Autodesk Fusion 360 part; units mm, degrees
(part 2 of 2)
sketch "USB B" plane through (0, 0, 0) normal (0, 1, 0) x (1, 0, 0) in component "USB"
  line L0 (7.35, -2.05) -> (7.35, 2.05)
  arc A0 (7.35, 2.05) -> (5.75, 3.65) centre (5.75, 2.05) ccw
  line L1 (5.75, 3.65) -> (-5.75, 3.65)
  arc A1 (-5.75, 3.65) -> (-7.35, 2.05) centre (-5.75, 2.05) ccw
  line L2 (-7.35, 2.05) -> (-7.35, -2.05)
  arc A2 (-7.35, -2.05) -> (-5.75, -3.65) centre (-5.75, -2.05) ccw
  line L3 (-5.75, -3.65) -> (5.75, -3.65)
  arc A3 (5.75, -3.65) -> (7.35, -2.05) centre (5.75, -2.05) ccw
  line L4 (0, 0) -> (-15, 0) construction
  circle A4 centre (-15, 0) radius 1.8
  circle A5 centre (15, 0) radius 1.8
  line L5 (7.35, 3.65) -> (-7.35, -3.65) construction
  line L6 (-7.35, 3.65) -> (7.35, -3.65) construction
  line L7 (20, 7.5) -> (-20, 7.5)
  line L8 (-20, 7.5) -> (-20, -7.5)
  line L9 (-20, -7.5) -> (20, -7.5)
  line L10 (20, -7.5) -> (20, 7.5)
  line L11 (20, 7.5) -> (-20, -7.5) construction
  line L12 (-20, 7.5) -> (20, -7.5) construction
  line L13 (0, -7.5) -> (0, 0) construction
  dimension "d555" = 14.7
  dimension "d556" = 7.3
  dimension "d557" = 1.6
  dimension "d558" = 1.6
  dimension "d559" = 1.6
  dimension "d560" = 1.6
  dimension "d561" = 15
  dimension "d562" = 3.6
  dimension "d240" = 15
  dimension "d241" = 40
  constraint horizontal L1
  constraint perpendicular L1 L2
  constraint parallel L1 L3
  constraint parallel L0 L2
  constraint coincident L6.start L1
  constraint coincident L6.start L2
  constraint tangent L1 A1
  constraint tangent A1 L2
  constraint coincident L5.start L0
  constraint coincident L5.start L1
  constraint tangent L0 A0
  constraint tangent A0 L1
  constraint coincident L6.end L0
  constraint coincident L6.end L3
  constraint tangent L0 A3
  constraint tangent L3 A3
  constraint coincident L5.end L2
  constraint coincident L5.end L3
  constraint tangent L2 A2
  constraint tangent A2 L3
  constraint perpendicular L2 L4
  constraint coincident L4.end A4.centre
  constraint horizontal L7
  constraint perpendicular L7 L8
  constraint parallel L7 L9
  constraint parallel L8 L10
  constraint coincident L11 L4.start
  constraint coincident L12 L4.start
  constraint coincident L4.start L13.end
  constraint midpoint L9 L13.start
  constraint symmetric A4 A5 L13
  measures "d555" distance of L5.end L6.end
  measures "d556" distance of L6.start L5.end
  measures "d557" radius of A1
  measures "d558" radius of A0
  measures "d559" radius of A3
  measures "d560" radius of A2
  measures "d561" distance of L4.end L4.start
  measures "d562" diameter of A4
  measures "d240" distance of L7.end L8.end
  measures "d241" distance of L8.end L9.end
sketch "RJ-45" plane through (0, 0, 0) normal (0, 1, 0) x (1, 0, 0) in component "Other Connectors"
  line L0 (0, -15.1) -> (0, 0)
  line L1 (0, 0) -> (17.8, 0)
  line L2 (17.8, 0) -> (17.8, -15.1)
  line L3 (17.8, -15.1) -> (0, -15.1)
  circle A0 centre (-4.6, -9.15) radius 1.675
  circle A1 centre (22.4, -9.15) radius 1.675
  line L4 (0, -15.1) -> (17.8, 0) construction
  line L5 (17.8, -15.1) -> (0, 0) construction
  line L6 (-4.6, -9.15) -> (22.4, -9.15) construction
  line L7 (8.9, -7.55) -> (8.9, -9.15) construction
  line L8 (26.4, 4.95) -> (-8.6, 4.95)
  line L9 (-8.6, 4.95) -> (-8.6, -20.05)
  line L10 (-8.6, -20.05) -> (26.4, -20.05)
  line L11 (26.4, -20.05) -> (26.4, 4.95)
  line L12 (26.4, 4.95) -> (-8.6, -20.05) construction
  line L13 (-8.6, 4.95) -> (26.4, -20.05) construction
  line L14 (8.9, -7.55) -> (14, -7.55) construction
  point P0 (8.9, -7.55)
  dimension "d596" = 3.35
  dimension "d597" = 3.35
  dimension "d244" = 1.6
  dimension "d245" = 15.1
  dimension "d246" = 17.8
  dimension "d247" = 27
  dimension "d248" = 35
  dimension "d249" = 25
  constraint coincident A0.centre L6.start
  constraint coincident A1.centre L6.end
  constraint perpendicular L2 L6
  constraint midpoint L5 P0
  constraint midpoint L6 L7.end
  constraint horizontal L8
  constraint perpendicular L8 L9
  constraint parallel L8 L10
  constraint parallel L9 L11
  constraint coincident L12 P0
  constraint coincident L13 P0
  constraint coincident P0 L7.start
  constraint perpendicular L7 L14
  constraint symmetric L8 L10 L14
  measures "d596" diameter of A0
  measures "d597" diameter of A1
  measures "d244" distance of P0 L7.end
  measures "d245" distance of L0.start L0.end
  measures "d246" distance of L2.end L0.start
  measures "d247" distance of A0.centre A1.centre
  measures "d248" distance of L9.end L10.end
  measures "d249" distance of L8.end L9.end
sketch "HDMI" plane through (0, 0, 0) normal (0, 1, 0) x (1, 0, 0) in component "Other Connectors"
  line L0 (-8.15, -3.0387) -> (-8.15, 1.8613)
  line L1 (-8.15, 1.8613) -> (-6.55, 1.8613)
  line L2 (-6.55, 1.8613) -> (-5.7382, 2.8326)
  line L3 (-5.7382, 2.8326) -> (0, 2.8326)
  line L4 (8.15, -3.0387) -> (-8.15, -3.0387)
  line L5 (8.15, -3.0387) -> (8.15, 1.8613)
  line L6 (8.15, 1.8613) -> (6.55, 1.8613)
  line L7 (6.55, 1.8613) -> (5.7382, 2.8326)
  line L8 (5.7382, 2.8326) -> (0, 2.8326)
  line L9 (0, 0) -> (13.25, 0) construction
  line L10 (0, 6) -> (0, -6) construction
  circle A0 centre (-13.25, 0) radius 1.8
  circle A1 centre (13.25, 0) radius 1.8
  line L11 (20, 6) -> (-20, 6)
  line L12 (-20, 6) -> (-20, -6)
  line L13 (-20, -6) -> (20, -6)
  line L14 (20, -6) -> (20, 6)
  dimension "d571" = 16.3
  dimension "d573" = 4.9
  dimension "d574" = 1.6
  dimension "d579" = 3.6
  dimension "d256" = 40
  dimension "d257" = 12
  constraint parallel L3 L4
  constraint coincident L3.end L10
  constraint coincident L9.end A1.centre
  constraint coincident L4.start L5
  constraint coincident L5.start L4
  constraint coincident L8.end L3
  constraint horizontal L9
  constraint horizontal L4
  constraint symmetric L10 A0 A1
  constraint symmetric L0 L5 L10
  constraint symmetric L2 L7 L10
  constraint symmetric L3 L8 L10
  constraint symmetric L10 L12 L14
  constraint symmetric L9 L11 L13
  measures "d571" distance of L4.start L0.start
  measures "d573" distance of L0.end L0.start
  measures "d574" distance of L0.end L1.end
  measures "d579" diameter of A1
  measures "d256" distance of L12.end L13.end
  measures "d257" distance of L12.end L11.end
sketch "40mm Fan Profile" plane through (0, 0, 0) normal (0, 1, 0) x (1, 0, 0) in component "Fans"
  circle A0 centre (0, 0) radius 19.5
  line L0 (16, 16) -> (-16, 16) construction
  line L1 (-16, 16) -> (-16, -16) construction
  line L2 (-16, -16) -> (16, -16) construction
  line L3 (16, -16) -> (16, 16) construction
  line L4 (16, 16) -> (-16, -16) construction
  line L5 (-16, 16) -> (16, -16) construction
  circle A1 centre (-16, 16) radius 1.8
  circle A2 centre (16, 16) radius 1.8
  circle A3 centre (-16, -16) radius 1.8
  circle A4 centre (16, -16) radius 1.8
  dimension "d258" = 39
  dimension "d259" = 32
  dimension "d260" = 32
  dimension "d261" = 3.6
  dimension "d262" = 3.6
  dimension "d263" = 3.6
  dimension "d264" = 3.6
  constraint coincident A0.centre origin
  constraint horizontal L0
  constraint perpendicular L0 L1
  constraint parallel L0 L2
  constraint parallel L1 L3
  constraint coincident L4 A0.centre
  constraint coincident L5 A0.centre
  constraint coincident L0.end L1.start
  constraint coincident L0.start L3.end
  constraint coincident L1.end L2.start
  constraint coincident L2.end L3.start
  measures "d258" diameter of A0
  measures "d259" distance of L1.end L2.end
  measures "d260" distance of L0.end L1.end
  measures "d261" diameter of A1
  measures "d262" diameter of A2
  measures "d263" diameter of A4
  measures "d264" diameter of A3
sketch "MF3 2R 14P" plane through (0, 0, 0) normal (0, 1, 0) x (1, 0, 0) in component "Molex Micro Fit 3"
  line L0 (-0.85, -4.975) -> (0.85, -3.575) construction
  line L1 (-11.075, 3.575) -> (11.075, -3.575) construction
  line L2 (0.85, -4.975) -> (-0.85, -3.575) construction
  line L3 (-13.25, 1.875) -> (13.25, -1.875) construction
  line L4 (-11.075, 3.575) -> (-11.075, -3.575) construction
  line L5 (0.85, -3.575) -> (11.075, -3.575)
  line L6 (11.075, 3.575) -> (-11.075, -3.575) construction
  line L7 (-0.85, -3.575) -> (-11.075, -3.575)
  line L8 (11.075, 3.575) -> (-11.075, 3.575)
  line L9 (0, -3.575) -> (0, -4.975) construction
  line L10 (-11.075, -3.575) -> (-11.075, -1.875)
  line L11 (0, -4.975) -> (0, 3.575) construction
  line L12 (14.75, 4.8) -> (14.75, -6.2)
  line L13 (13.25, 1.875) -> (-13.25, -1.875) construction
  line L14 (0.85, -4.975) -> (-0.85, -4.975)
  line L15 (-14.75, -6.2) -> (-14.75, 4.8)
  line L16 (-14.75, 4.8) -> (14.75, 4.8)
  line L17 (11.075, 1.875) -> (11.075, 3.575)
  line L18 (-11.075, -1.875) -> (-13.25, -1.875)
  line L19 (11.075, 1.875) -> (13.25, 1.875)
  line L20 (11.075, -1.875) -> (13.25, -1.875)
  line L21 (11.075, -3.575) -> (11.075, 3.575) construction
  line L22 (0.85, -3.575) -> (0.85, -4.975)
  line L23 (-13.25, 1.875) -> (-13.25, -1.875)
  line L24 (13.25, -1.875) -> (13.25, 1.875)
  line L25 (-11.075, 1.875) -> (-11.075, 3.575)
  line L26 (-0.85, -4.975) -> (-0.85, -3.575)
  line L27 (-13.25, 1.875) -> (-11.075, 1.875)
  line L28 (-11.075, -3.575) -> (11.075, -3.575) construction
  line L29 (13.25, 1.875) -> (-13.25, 1.875) construction
  line L30 (11.075, -3.575) -> (11.075, -1.875)
  line L31 (-13.25, -1.875) -> (13.25, -1.875) construction
  line L32 (-0.85, -3.575) -> (0.85, -3.575) construction
  line L33 (14.75, -6.2) -> (-14.75, -6.2)
  line L34 (14.75, -6.2) -> (-14.75, 4.8) construction
  line L35 (-14.75, -6.2) -> (14.75, 4.8) construction
  point P0 (-3, 0)
  point P1 (0, -0.7)
  point P2 (0, -4.275)
  dimension "d330" = 22.15
  dimension "d331" = 7.15
  dimension "d332" = 26.5
  dimension "d333" = 3.75
  dimension "d334" = 1.4
  dimension "d335" = 1.7
  dimension "d336" = 29.5
  dimension "d337" = 11
  constraint horizontal L8
  constraint perpendicular L4 L8
  constraint parallel L8 L28
  constraint parallel L4 L21
  constraint coincident origin L6
  constraint coincident origin L1
  constraint horizontal L29
  constraint perpendicular L23 L29
  constraint parallel L29 L31
  constraint parallel L23 L24
  constraint coincident origin L13
  constraint coincident origin L3
  constraint midpoint L9.start L28
  constraint perpendicular L9 L28
  constraint horizontal L14
  constraint perpendicular L14 L26
  constraint parallel L14 L32
  constraint parallel L22 L26
  constraint coincident P2 L2
  constraint coincident P2 L0
  constraint midpoint P2 L9
  constraint perpendicular L4 L7
  constraint coincident L10.end L31
  constraint coincident L10.end L4
  constraint coincident L25.start L29
  constraint coincident L25.start L4
  constraint coincident L17.start L29
  constraint coincident L17.start L21
  constraint coincident L20.start L21
  constraint coincident L20.start L31
  constraint midpoint L11.end L8
  constraint horizontal L33
  constraint perpendicular L15 L33
  constraint parallel L16 L33
  constraint parallel L12 L15
  constraint coincident P1 L34
  constraint coincident P1 L35
  constraint midpoint P1 L11
  measures "d330" distance of L4.end L1.end
  measures "d331" distance of L1.start L4.end
  measures "d332" distance of L13.end L3.end
  measures "d333" distance of L13.end L3.start
  measures "d334" distance of L9.start L9.end
  measures "d335" distance of L0.end L2.end
  measures "d336" distance of L15.start L12.end
  measures "d337" distance of L15.start L15.end
extrude "Extrude1" add sketch "MF3 1R 2P" along normal blind 1.8 makes body 1 in component "MF3 1R 2P"
extrude "Extrude1'" add sketch "MF3 1R 3P" along normal blind 1.8 separate body makes body 2 in component "MF3 1R 3P"
extrude "Extrude1''" add sketch "MF3 1R 4P" along normal blind 1.8 separate body makes body 3 in component "MF3 1R 4P"
extrude "Extrude1'''" add sketch "MF3 1R 5P" along normal blind 1.8 separate body makes body 4 in component "MF3 1R 5P"
extrude "Extrude1''''" add sketch "MF3 2R 2P" along normal blind 1.8 separate body makes body 5 in component "MF3 2R 2P"
extrude "Extrude1'''''" add sketch "MF3 2R 4P" along normal blind 1.8 separate body makes body 6 in component "MF3 2R 4P"
extrude "Extrude1''''''" add sketch "MF3 2R 6P" along normal blind 2.4 separate body makes body 7 in component "MF3 2R 6P"
extrude "Extrude1'''''''" add sketch "MF3 2R 8P" along normal blind 1.8 separate body makes body 8 in component "MF3 2R 8P"
extrude "Extrude1''''''''" add sketch "MF3 2R 10P" along normal blind 2.4 separate body makes body 9 in component "MF3 2R 10P"
extrude "Extrude1'''''''''" add sketch "MF3 2R 12P" along normal blind 2.4 separate body makes body 10 in component "MF3 2R 12P"
extrude "Extrude1''''''''''" add sketch "MF3 2R 14P" along normal blind 2.4 separate body makes body 11 in component "MF3 2R 14P"
extrude "Extrude1'''''''''''" add sketch "MF3 2R 16P" along normal blind 1.8 separate body makes body 12 in component "MF3 2R 16P"
sketch "USB Logo" plane through (0, 0, 0) normal (0, 1, 0) x (1, 0, 0) in component "USB"
  spline S0 degree 3 poles (-0.5083, -3.738) (-0.113, -4.1192) (0.5084, -4.4442) (1.1013, -4.4442) knots 0 0 0 0 1 1 1 1
  line L0 (1.1013, -4.4442) -> (3.2091, -4.4437)
  line L1 (3.2091, -4.4437) -> (3.2091, -5.3315)
  line L2 (3.2091, -5.3315) -> (5.8576, -5.3315)
  line L3 (5.8576, -5.3315) -> (5.8576, -2.6833)
  line L4 (5.8576, -2.6833) -> (3.2091, -2.6833)
  line L5 (3.2091, -2.6833) -> (3.2091, -3.5699)
  spline S1 degree 2 poles (3.2091, -3.5699) (2.6539, -3.5689) (1.0755, -3.5689) knots 0 0 0 1 1 1
  spline S2 degree 3 poles (1.0755, -3.5689) (0.7736, -3.562) (0.4799, -3.436) (0.2557, -3.2563) knots 0 0 0 0 1 1 1 1
  line L6 (0.2557, -3.2563) -> (-2.38, -0.4717)
  line L7 (-2.38, -0.4717) -> (7.8439, -0.4717)
  line L8 (7.8439, -0.4717) -> (7.8439, -1.5642)
  line L9 (7.8439, -1.5642) -> (10.4917, -0.0354)
  line L10 (10.4917, -0.0354) -> (7.8439, 1.4937)
  line L11 (7.8439, 1.4937) -> (7.8439, 0.403)
  line L12 (7.8439, 0.403) -> (-5.6896, 0.403)
  line L13 (-5.6896, 0.403) -> (-3.0545, 3.187)
  spline S3 degree 3 poles (-3.0545, 3.187) (-2.8302, 3.3668) (-2.5368, 3.4929) (-2.235, 3.4998) knots 0 0 0 0 1 1 1 1
  spline S4 degree 3 poles (-2.235, 3.4998) (-1.0139, 3.4998) (-0.2888, 3.5002) (-0.0219, 3.5007) knots 0 0 0 0 1 1 1 1
  spline S5 degree 3 poles (-0.0219, 3.5007) (0.159, 2.9852) (0.645, 2.6132) (1.2227, 2.6132) knots 0 0 0 0 1 1 1 1
  spline S6 degree 3 poles (1.2227, 2.6132) (1.9536, 2.6132) (2.5468, 3.2063) (2.5468, 3.9374) knots 0 0 0 0 1 1 1 1
  spline S7 degree 3 poles (2.5468, 3.9374) (2.5468, 4.6689) (1.9537, 5.2618) (1.2227, 5.2618) knots 0 0 0 0 1 1 1 1
  spline S8 degree 3 poles (1.2227, 5.2618) (0.645, 5.2618) (0.159, 4.8899) (-0.0219, 4.3749) knots 0 0 0 0 1 1 1 1
  line L14 (-0.0219, 4.3749) -> (-2.2091, 4.3752)
  spline S9 degree 3 poles (-2.2091, 4.3752) (-2.8018, 4.3752) (-3.423, 4.05) (-3.8183, 3.6688) knots 0 0 0 0 1 1 1 1
  spline S10 degree 3 poles (-3.8183, 3.6688) (-3.8075, 3.6801) (-3.7963, 3.6921) (-3.8189, 3.6685) knots 0 0 0 0 1 1 1 1
  spline S11 degree 2 poles (-3.8189, 3.6685) (-3.8273, 3.6591) (-6.6147, 0.7151) knots 0 0 0 1 1 1
  spline S12 degree 3 poles (-6.6147, 0.7151) (-6.8385, 0.5356) (-7.1318, 0.4103) (-7.4334, 0.4031) knots 0 0 0 0 1 1 1 1
  line L15 (-7.4334, 0.4031) -> (-8.9644, 0.4031)
  spline S13 degree 3 poles (-8.9644, 0.4031) (-9.1673, 1.4145) (-10.0605, 2.1765) (-11.1318, 2.1765) knots 0 0 0 0 1 1 1 1
  spline S14 degree 3 poles (-11.1318, 2.1765) (-12.3533, 2.1765) (-13.3434, 1.1863) (-13.3434, -0.0348) knots 0 0 0 0 1 1 1 1
  spline S15 degree 3 poles (-13.3434, -0.0348) (-13.3434, -1.2563) (-12.3533, -2.2464) (-11.1318, -2.2464) knots 0 0 0 0 1 1 1 1
  spline S16 degree 3 poles (-11.1318, -2.2464) (-10.0602, -2.2464) (-9.1671, -1.4838) (-8.9642, -0.4715) knots 0 0 0 0 1 1 1 1
  line L16 (-8.9642, -0.4715) -> (-7.46, -0.4715)
  spline S17 degree 3 poles (-7.46, -0.4715) (-7.4562, -0.4715) (-7.4523, -0.4718) (-7.4484, -0.4715) knots 0 0 0 0 1 1 1 1
  line L17 (-7.4484, -0.4715) -> (-4.1215, -0.4715)
  spline S18 degree 3 poles (-4.1215, -0.4715) (-3.8204, -0.4792) (-3.5275, -0.6047) (-3.304, -0.7844) knots 0 0 0 0 1 1 1 1
  spline S19 degree 2 poles (-3.304, -0.7844) (-0.5172, -3.7283) (-0.5085, -3.7378) knots 0 0 0 1 1 1
  spline S20 degree 3 poles (-0.5085, -3.7378) (-0.4862, -3.7614) (-0.4973, -3.7491) (-0.5083, -3.738) knots 0 0 0 0 1 1 1 1
extrude "Extrude1''''''''''''" add sketch "JST SM 2P" along normal blind 2 separate body makes body 13 in component "JST SM 2P"
extrude "Extrude1'''''''''''''" add sketch "JST SM 3P" along normal blind 2 separate body makes body 14 in component "JST SM 3P"
extrude "Extrude1''''''''''''''" add sketch "JST SM 4P" along normal blind 2 separate body makes body 15 in component "JST SM 4P"
extrude "Extrude1'''''''''''''''" add sketch "JST SM 5P" along normal blind 2 separate body makes body 16 in component "JST SM 5P"
extrude "Extrude1''''''''''''''''" add sketch "RJ-45" along normal blind 2 separate body makes body 17 in component "RJ-45"
extrude "Extrude1'''''''''''''''''" add sketch "HDMI" along normal blind 2 separate body makes body 18 in component "HDMI"
extrude "Extrude1''''''''''''''''''" add sketch "USB-C" along normal blind 2 separate body makes body 19 in component "USB-C"
extrude "Extrude1'''''''''''''''''''" add sketch "USB A" along normal blind 2 separate body makes body 20 in component "USB A"
extrude "Extrude1''''''''''''''''''''" add sketch "USB B" along normal blind 2 separate body makes body 21 in component "USB B"
sketch "92mm Fan Profile" plane through (0, 0, 0) normal (0, 1, 0) x (1, 0, 0) in component "Fans"
  circle A0 centre (0, 0) radius 45.5
  line L0 (41.25, 41.25) -> (-41.25, -41.25) construction
  line L1 (-41.25, 41.25) -> (41.25, -41.25) construction
  circle A1 centre (-41.25, 41.25) radius 2.3
  circle A2 centre (41.25, 41.25) radius 2.3
  circle A3 centre (41.25, -41.25) radius 2.3
  circle A4 centre (-41.25, -41.25) radius 2.3
  dimension "d346" = 91
  dimension "d347" = 82.5
  dimension "d348" = 82.5
  dimension "d349" = 4.6
  dimension "d350" = 4.6
  dimension "d351" = 4.6
  dimension "d352" = 4.6
  constraint coincident A0.centre origin
  constraint coincident L0 A0.centre
  constraint coincident L1 A0.centre
  constraint coincident L1.start A1.centre
  constraint coincident L0.start A2.centre
  constraint coincident L1.end A3.centre
  constraint coincident L0.end A4.centre
  measures "d346" diameter of A0
  measures "d347" distance of L0.end L1.end
  measures "d348" distance of L1.start L0.end
  measures "d349" diameter of A4
  measures "d350" diameter of A3
  measures "d351" diameter of A2
  measures "d352" diameter of A1
sketch "XT60" plane through (0, 0, 0) normal (0, 1, 0) x (1, 0, 0) in component "Other Connectors"
  line L0 (-4.025, -4.75) -> (-4.025, 7.75) construction
  line L1 (0, -7.75) -> (0, -10.25) construction
  arc A0 (-4.025, -4.75) -> (-1.025, -7.75) centre (-1.025, -4.75) ccw construction
  line L2 (-4.025, 7.75) -> (4.025, -7.75) construction
  circle A1 centre (0, -10.25) radius 1.65
  line L3 (-4.175, -4.75) -> (-4.175, 7.9)
  line L4 (4.025, 7.75) -> (-4.025, -7.75) construction
  line L5 (6, 14) -> (-6, -14) construction
  line L6 (-4.025, 7.75) -> (4.025, 7.75) construction
  circle A2 centre (0, 10.25) radius 1.65
  line L7 (6, -14) -> (-6, -14)
  line L8 (-6, 14) -> (6, 14)
  line L9 (-4.175, 7.9) -> (4.175, 7.9)
  line L10 (6, 14) -> (6, -14)
  line L11 (1.025, -7.9) -> (-1.025, -7.9)
  line L12 (0, 7.75) -> (0, 10.25) construction
  line L13 (-6, 14) -> (6, -14) construction
  line L14 (1.025, -7.75) -> (-1.025, -7.75) construction
  arc A3 (1.025, -7.75) -> (4.025, -4.75) centre (1.025, -4.75) ccw construction
  line L15 (4.175, 7.9) -> (4.175, -4.75)
  line L16 (-6, -14) -> (-6, 14)
  arc A4 (-4.175, -4.75) -> (-1.025, -7.9) centre (-1.025, -4.75) ccw
  arc A5 (1.025, -7.9) -> (4.175, -4.75) centre (1.025, -4.75) ccw
  line L17 (4.025, 7.75) -> (4.025, -4.75) construction
  dimension "d1" = 15.5
  dimension "d2" = 8.05
  dimension "d3" = 3
  dimension "d4" = 3
  dimension "d5" = 2.5
  dimension "d6" = 3.3
  dimension "d7" = 2.5
  dimension "d8" = 3.3
  dimension "d11" = 12
  dimension "d12" = 28
  constraint perpendicular L6 L17
  constraint parallel L6 L14
  constraint parallel L0 L17
  constraint coincident origin L2
  constraint coincident origin L4
  constraint coincident L2.end L17
  constraint coincident L2.end L14
  constraint tangent A3 L17
  constraint tangent L14 A3
  constraint coincident L4.end L14
  constraint coincident L4.end L0
  constraint tangent A0 L14
  constraint tangent L0 A0
  constraint midpoint L12.start L6
  constraint perpendicular L6 L12
  constraint coincident A2.centre L12.end
  constraint midpoint L1.start L14
  constraint perpendicular L1 L14
  constraint coincident L1.end A1.centre
  constraint perpendicular L8 L10
  constraint parallel L7 L8
  constraint parallel L10 L16
  constraint coincident origin L13
  constraint coincident origin L5
  constraint concentric A3 A5
  constraint concentric A0 A4
  constraint tangent L15 A5
  constraint tangent L11 A5
  constraint tangent L3 A4
  constraint tangent L11 A4
  measures "d1" distance of L2.end L4.start
  measures "d2" distance of L2.end L4.end
  measures "d3" radius of A3
  measures "d4" radius of A0
  measures "d5" distance of A2.centre L12.start
  measures "d6" diameter of A2
  measures "d7" distance of L1.start L1.end
  measures "d8" diameter of A1
  measures "d11" distance of L5.end L7.start
  measures "d12" distance of L5.start L7.start
extrude "Extrude1'''''''''''''''''''''" add sketch "XT60" along normal blind 3 separate body makes body 22 in component "XT60"
sketch "2R 2P" plane through (0, 0, 0) normal (0, 1, 0) x (1, 0, 0) in component "Molex Mini Fit Jr"
  line L0 (3.1, 5.4) -> (0, 5.4)
  line L1 (3.1, -4.6) -> (3.1, 5.4) construction
  line L2 (5.4, 2.9) -> (3.1, 2.9)
  line L3 (3.1, -4.6) -> (3.1, -2.5)
  line L4 (-3.1, 5.4) -> (0, 5.4)
  line L5 (-3.1, -4.6) -> (-3.1, -2.5)
  line L6 (7, 7.8) -> (-7, -8.2) construction
  line L7 (-5.4, -2.5) -> (-3.1, -2.5)
  line L8 (-5.4, 2.9) -> (-3.1, 2.9)
  line L9 (-7, 7.8) -> (7, -8.2) construction
  line L10 (1.9, -4.6) -> (3.1, -4.6)
  line L11 (-1.9, -6.2) -> (-1.9, -4.6)
  line L12 (-7, 7.8) -> (7, 7.8)
  line L13 (0, -6.2) -> (0, 5.4) construction
  line L14 (5.4, 2.9) -> (5.4, -2.5)
  line L15 (1.9, -4.6) -> (-3.1, -4.6) construction
  line L16 (0, -6.2) -> (1.9, -6.2)
  line L17 (-7, -8.2) -> (-7, 7.8)
  line L18 (1.9, -6.2) -> (1.9, -4.6)
  line L19 (5.4, -2.5) -> (3.1, -2.5)
  line L20 (0, -4.6) -> (3.1, -4.6) construction
  line L21 (-3.1, 2.9) -> (-3.1, 5.4)
  line L22 (3.1, 0.4) -> (5.1, 0.4) construction
  line L23 (7, 7.8) -> (7, -8.2)
  line L24 (7, -8.2) -> (-7, -8.2)
  line L25 (-1.9, -4.6) -> (-3.1, -4.6)
  line L26 (-5.4, 2.9) -> (-5.4, -2.5)
  line L27 (3.1, 2.9) -> (3.1, 5.4)
  line L28 (0, -6.2) -> (-1.9, -6.2)
  point P0 (0, -0.2)
  point P1 (0, -0.2)
  point P2 (0, 6)
  dimension "d19" = 2
  dimension "d23" = 1.9
  dimension "d368" = 1.6
  dimension "d369" = 1.2
  dimension "d370" = 10
  dimension "d371" = 14
  dimension "d372" = 16
  dimension "d35" = 2.3
  dimension "d36" = 5.4
  dimension "d37" = 2.5
  dimension "d38" = 2.1
  constraint coincident L15.start L10
  constraint coincident L10.start L18
  constraint perpendicular L1 L20
  constraint midpoint L22.start L1
  constraint perpendicular L1 L22
  constraint coincident L2.end L1
  constraint coincident L3.end L1
  constraint perpendicular L0 L27
  constraint perpendicular L0 L13
  constraint coincident L20.start L13
  constraint symmetric L5.start L1.start L13
  constraint perpendicular L12 L23
  constraint parallel L12 L24
  constraint parallel L17 L23
  constraint coincident P1 L9
  constraint coincident P1 L6
  constraint coincident P1 P0
  constraint perpendicular L2 L27
  constraint perpendicular L3 L19
  constraint symmetric L10.start L11.end L13
  constraint symmetric L1.start L5.start L13
  constraint symmetric L0.start L4.start L13
  constraint symmetric L16.end L11.start L13
  constraint symmetric L2.start L8.start L13
  constraint symmetric L14.end L7.start L13
  constraint symmetric L2.end L8.end L13
  constraint symmetric L3.end L5.end L13
  constraint symmetric L16.start L28.start L13
  constraint symmetric L0.end L4.end L13
  constraint coincident P1 L13
  measures "d19" distance of L22.start L22.end
  measures "d23" distance of L13.start L16.end
  measures "d368" distance of L10.start L16.end
  measures "d369" distance of L1 L18
  measures "d370" distance of L0.start L1.start
  measures "d371" distance of L9.end L6.end
  measures "d372" distance of L6.start L9.end
  measures "d35" distance of L14.end L3.end
  measures "d36" distance of L14.end L2.start
  measures "d37" distance of L0.start L2
  measures "d38" distance of L1.start L19
extrude "Extrude1''''''''''''''''''''''" add sketch "2R 2P" along normal blind 1.6 separate body makes body 23 in component "Mini Fit Jr 2R 2P"
sketch "IEC C13" plane through (0, 0, 0) normal (0, 1, 0) x (1, 0, 0) in component "Other Connectors"
  arc A0 (-35.25, -32.2) -> (-33, -34.45) centre (-33, -32.2) ccw
  line L0 (-35.25, -32.2) -> (-35.25, -11.5745)
  arc A1 (-34.6539, -10.0491) -> (-35.25, -11.5745) centre (-33, -11.5745) ccw
  line L1 (-28.7744, -3.6745) -> (-34.6539, -10.0491)
  arc A2 (-27.1205, -2.95) -> (-28.7744, -3.6745) centre (-27.1205, -5.2) ccw
  line L2 (-27.1205, -2.95) -> (-15.8795, -2.95)
  arc A3 (-14.2456, -3.6531) -> (-15.8795, -2.95) centre (-15.8795, -5.2) ccw
  line L3 (-8.3661, -9.8633) -> (-14.2456, -3.6531)
  arc A4 (-7.75, -11.4102) -> (-8.3661, -9.8633) centre (-10, -11.4102) ccw
  line L4 (-7.75, -11.4102) -> (-7.75, -32.2)
  arc A5 (-10, -34.45) -> (-7.75, -32.2) centre (-10, -32.2) ccw
  line L5 (-10, -34.45) -> (-33, -34.45)
  line L6 (-21.5, -2.95) -> (-21.5, -34.45) construction
  line L7 (-3.5, -18.7) -> (-39.5, -18.7) construction
  circle A6 centre (-39.5, -18.7) radius 1.4
  circle A7 centre (-3.5, -18.7) radius 1.4
  line L8 (0, -0.2) -> (-43, -0.2)
  line L9 (-43, -0.2) -> (-43, -37.2)
  line L10 (-43, -37.2) -> (0, -37.2)
  line L11 (0, -37.2) -> (0, -0.2)
  line L12 (0, -0.2) -> (-43, -37.2) construction
  line L13 (-43, -0.2) -> (0, -37.2) construction
  point P0 (-21.5, -18.7)
  dimension "d79" = 2.8
  dimension "d380" = 2.25
  dimension "d381" = 2.25
  dimension "d382" = 2.25
  dimension "d221" = 2.25
  dimension "d384" = 2.25
  dimension "d385" = 2.25
  dimension "d386" = 31.5
  dimension "d387" = 27.5
  dimension "d388" = 15.75
  dimension "d389" = 36
  dimension "d390" = 2.8
  dimension "d391" = 43
  dimension "d392" = 37
  constraint coincident L7.start A7.centre
  constraint coincident L7.end A6.centre
  constraint perpendicular L0 L7
  constraint midpoint L6.start L2
  constraint midpoint L6.end L5
  constraint perpendicular L5 L6
  constraint midpoint L6 L7
  constraint horizontal L2
  constraint tangent A5 L5
  constraint tangent A0 L5
  constraint tangent A0 L0
  constraint tangent L0 A1
  constraint tangent A1 L1
  constraint tangent L1 A2
  constraint tangent A2 L2
  constraint tangent L2 A3
  constraint tangent A3 L3
  constraint tangent L3 A4
  constraint tangent A4 L4
  constraint tangent L4 A5
  constraint horizontal L8
  constraint perpendicular L8 L9
  constraint parallel L8 L10
  constraint parallel L9 L11
  constraint coincident L12 P0
  constraint coincident L13 P0
  constraint midpoint L6 P0
  measures "d79" diameter of A6
  measures "d380" radius of A0
  measures "d381" radius of A5
  measures "d382" radius of A4
  measures "d221" radius of A3
  measures "d384" radius of A1
  measures "d385" radius of A2
  measures "d386" distance of L2 L5
  measures "d387" distance of L0 L4
  measures "d388" distance of L5 L7
  measures "d389" distance of L7.end L7.start
  measures "d390" diameter of A7
  measures "d391" distance of L9.end L10.end
  measures "d392" distance of L8.end L9.end
extrude "Extrude1'''''''''''''''''''''''" add sketch "IEC C13" along normal blind 5 separate body makes body 24 in component "IEC C13 Socket"
component "Molex Micro Fit 3" placed x (1, 0, 0) y (0, 1, 0) z (0, 0, 1) at (0, 0, 0)
component "Fans" placed x (1, 0, 0) y (0, 1, 0) z (0, 0, 1) at (0, 0, 0)
component "USB" placed x (1, 0, 0) y (0, 1, 0) z (0, 0, 1) at (0, 0, 0)
component "JST SM" placed x (1, 0, 0) y (0, 1, 0) z (0, 0, 1) at (0, 0, 0)
component "Other Connectors" placed x (1, 0, 0) y (0, 1, 0) z (0, 0, 1) at (0, 0, 0)
component "Molex Mini Fit Jr" placed x (1, 0, 0) y (0, 1, 0) z (0, 0, 1) at (0, 0, 0)
component "MF3 1R 2P" placed x (1, 0, 0) y (0, 1, 0) z (0, 0, 1) at (0, 0, 0) in component "Molex Micro Fit 3"
component "MF3 1R 3P" placed x (1, 0, 0) y (0, 1, 0) z (0, 0, 1) at (0, 0, 0) in component "Molex Micro Fit 3"
component "MF3 1R 4P" placed x (1, 0, 0) y (0, 1, 0) z (0, 0, 1) at (0, 0, 0) in component "Molex Micro Fit 3"
component "MF3 1R 5P" placed x (1, 0, 0) y (0, 1, 0) z (0, 0, 1) at (0, 0, 0) in component "Molex Micro Fit 3"
component "MF3 2R 2P" placed x (1, 0, 0) y (0, 1, 0) z (0, 0, 1) at (0, 0, 0) in component "Molex Micro Fit 3"
component "MF3 2R 4P" placed x (1, 0, 0) y (0, 1, 0) z (0, 0, 1) at (0, 0, 0) in component "Molex Micro Fit 3"
component "MF3 2R 6P" placed x (1, 0, 0) y (0, 1, 0) z (0, 0, 1) at (0, 0, 0) in component "Molex Micro Fit 3"
component "MF3 2R 8P" placed x (1, 0, 0) y (0, 1, 0) z (0, 0, 1) at (0, 0, 0) in component "Molex Micro Fit 3"
component "MF3 2R 10P" placed x (1, 0, 0) y (0, 1, 0) z (0, 0, 1) at (0, 0, 0) in component "Molex Micro Fit 3"
component "MF3 2R 12P" placed x (1, 0, 0) y (0, 1, 0) z (0, 0, 1) at (0, 0, 0) in component "Molex Micro Fit 3"
component "MF3 2R 14P" placed x (1, 0, 0) y (0, 1, 0) z (0, 0, 1) at (0, 0, 0) in component "Molex Micro Fit 3"
component "MF3 2R 16P" placed x (1, 0, 0) y (0, 1, 0) z (0, 0, 1) at (0, 0, 0) in component "Molex Micro Fit 3"
component "USB-C" placed x (1, 0, 0) y (0, 1, 0) z (0, 0, 1) at (0, 0, 0) in component "USB"
component "USB A" placed x (1, 0, 0) y (0, 1, 0) z (0, 0, 1) at (0, 0, 0) in component "USB"
component "USB B" placed x (1, 0, 0) y (0, 1, 0) z (0, 0, 1) at (0, 0, 0) in component "USB"
component "JST SM 2P" placed x (1, 0, 0) y (0, 1, 0) z (0, 0, 1) at (0, 0, 0) in component "JST SM"
component "JST SM 3P" placed x (1, 0, 0) y (0, 1, 0) z (0, 0, 1) at (0, 0, 0) in component "JST SM"
component "JST SM 4P" placed x (1, 0, 0) y (0, 1, 0) z (0, 0, 1) at (0, 0, 0) in component "JST SM"
component "JST SM 5P" placed x (1, 0, 0) y (0, 1, 0) z (0, 0, 1) at (0, 0, 0) in component "JST SM"
component "RJ-45" placed x (1, 0, 0) y (0, 1, 0) z (0, 0, 1) at (0, 0, 0) in component "Other Connectors"
component "HDMI" placed x (1, 0, 0) y (0, 1, 0) z (0, 0, 1) at (0, 0, 0) in component "Other Connectors"
component "XT60" placed x (1, 0, 0) y (0, 1, 0) z (0, 0, 1) at (0, 0, 0) in component "Other Connectors"
component "IEC C13 Socket" placed x (1, 0, 0) y (0, 1, 0) z (0, 0, 1) at (0, 0, 0) in component "Other Connectors"
component "Mini Fit Jr 2R 2P" placed x (1, 0, 0) y (0, 1, 0) z (0, 0, 1) at (0, 0, 0) in component "Molex Mini Fit Jr"
equation "d96 = mf3_1r_clip_w + ( 3 * 3 ) * 1 mm"
equation "d97 = mf3_1r_clip_h"
equation "d98 = d96 + 3 mm"
equation "d105 = d162 + 3 mm"
equation "mf3_1r_clip_h = 3.15 mm" comment "1 Row Clip Height"
equation "mf3_1r_key_h = 1.2 mm" comment "1 Row Key Height"
equation "mf3_1r_base_h = 3 mm + mf3_base_calc" comment "1 Row Base Rect Height"
equation "mf3_pin_w = 3 mm" comment "Pin Hole Rect Width"
equation "mf3_pin_h = 3 mm" comment "Pin Hole Rect Height"
equation "mf3_base_calc = 1.15 mm" comment "Base Rect Calculated Dimension w/o Pins"
equation "mf3_1r_clip_w = 5.5 mm" comment "1 Row Clip Width w/o Pins"
equation "mf3_1r_key_w = 2.9 mm" comment "1 Row Key Width"
equation "d120 = mf3_base_calc + ( 4 * 3 ) * 1 mm"
equation "d121 = mf3_1r_base_h"
equation "d122 = mf3_1r_key_h"
equation "d123 = mf3_1r_key_w"
equation "d124 = mf3_1r_clip_w + ( 3 * 4 ) * 1 mm"
equation "d125 = mf3_1r_clip_h"
equation "d128 = d124 + 4 mm"
equation "d129 = mf3_1r_key_h"
equation "d130 = mf3_1r_key_w"
equation "d131 = mf3_1r_base_h"
equation "d132 = mf3_base_calc + ( 3 * 3 ) * 1 mm"
equation "d134 = mf3_1r_clip_w + ( 5 * 3 ) * 1 mm"
equation "d135 = mf3_1r_clip_h"
equation "d136 = mf3_base_calc + ( 3 * 5 ) * 1 mm"
equation "d137 = mf3_1r_base_h"
equation "d138 = mf3_1r_key_h"
equation "d139 = mf3_1r_key_w"
equation "d140 = mf3_1r_key_h"
equation "d142 = d134 + 2 mm"
equation "mf3_2r_key_h = 1.4 mm" comment "2 Row Key Height"
equation "mf3_2r_key_w = 1.7 mm" comment "2 Row Key Width"
equation "mf3_2r_clip_w = 5.5 mm" comment "2 Row Clip Width w/o Pins"
equation "mf3_2r_clip_h = 3.75 mm" comment "2 Row Clip Height"
equation "mf3_2r_base_h = ( 2 * 3 ) * 1 mm + mf3_base_calc" comment "2 Row Base Rect Height"
equation "d162 = mf3_1r_clip_w + 3 mm"
equation "d163 = mf3_2r_clip_h"
equation "d164 = mf3_base_calc + 3 mm"
equation "d165 = mf3_2r_base_h"
equation "d166 = mf3_1r_key_h"
equation "d167 = mf3_2r_key_w"
equation "d176 = mf3_base_calc + 6 mm"
equation "d177 = mf3_base_calc * 6"
equation "d178 = mf3_1r_clip_w + 6 mm"
equation "d179 = mf3_2r_clip_h"
equation "d180 = mf3_2r_key_h"
equation "d181 = mf3_2r_key_w"
equation "d185 = d178 + 3 mm"
equation "d186 = mf3_base_calc + ( 3 * 4 ) * 1 mm"
equation "d187 = mf3_2r_base_h"
equation "d188 = mf3_1r_clip_w + ( 3 * 4 ) * 1 mm"
equation "d189 = mf3_2r_clip_h"
equation "d190 = mf3_2r_key_h"
equation "d191 = mf3_2r_key_w"
equation "d192 = d188 + 3 mm"
equation "d194 = mf3_2r_clip_w + ( 3 * 8 ) * 1 mm"
equation "d195 = mf3_2r_clip_h"
equation "d196 = mf3_base_calc + ( 3 * 8 ) * 1 mm"
equation "d197 = mf3_2r_base_h"
equation "d198 = mf3_2r_key_h"
equation "d199 = mf3_2r_key_w"
equation "d201 = d194 + 3 mm"
equation "d218 = fan_hole_dia"
equation "d219 = fan_hole_dia"
equation "d220 = fan_hole_dia"
equation "fan_hole_dia = 3.6 mm" comment "Through hole diameter for fans"
equation "d222 = fan_hole_dia"
equation "d223 = mf3_1r_clip_w + 6 mm"
equation "d224 = mf3_1r_clip_h"
equation "d225 = mf3_base_calc + 6 mm"
equation "d226 = mf3_1r_base_h"
equation "d227 = mf3_1r_key_h"
equation "d228 = mf3_1r_key_w"
equation "d229 = d223 + 3 mm"
equation "d558 = d557"
equation "d559 = d557"
equation "d560 = d557"
equation "d596 = M3_hole_dia_Ref"
equation "d597 = M3_hole_dia_Ref"
equation "d262 = d261"
equation "d263 = d261"
equation "d264 = d261"
equation "d265 = mf3_depth"
equation "d267 = mf3_depth"
equation "d269 = mf3_depth"
equation "d271 = mf3_depth"
equation "d273 = mf3_depth"
equation "d275 = mf3_depth"
equation "d277 = mf3_depth"
equation "d279 = mf3_depth"
equation "d281 = jst_sm_depth"
equation "mf3_depth = 1.8 mm" comment "Depth of Micro Fit 3 panel mount"
equation "jst_sm_depth = 2 mm" comment "Depth for JST SM panel mounts"
equation "d287 = jst_sm_depth"
equation "d289 = jst_sm_depth"
equation "d291 = jst_sm_depth"
equation "d305 = mf3_base_calc + ( 3 * 3 ) * 1 mm"
equation "d306 = mf3_2r_base_h"
equation "d307 = mf3_2r_clip_w + 9 mm"
equation "d308 = mf3_2r_clip_h"
equation "d309 = mf3_2r_key_h"
equation "d310 = mf3_2r_key_w"
equation "d312 = d307 + 3 mm"
equation "d314 = mf3_base_calc + ( 3 * 5 ) * 1 mm"
equation "d315 = mf3_2r_base_h"
equation "d316 = mf3_2r_clip_w + 3 * 5 mm"
equation "d317 = mf3_2r_clip_h"
equation "d318 = mf3_2r_key_h"
equation "d319 = mf3_2r_key_w"
equation "d320 = d316 + 3 mm"
equation "d322 = mf3_base_calc + ( 3 * 6 ) * 1 mm"
equation "d323 = mf3_2r_base_h"
equation "d324 = mf3_2r_clip_w + 3 * 6 mm"
equation "d325 = mf3_2r_clip_h"
equation "d326 = mf3_2r_key_h"
equation "d327 = mf3_2r_key_w"
equation "d328 = d324 + 3 mm"
equation "d330 = mf3_base_calc + ( 3 * 7 ) * 1 mm"
equation "d331 = mf3_2r_base_h"
equation "d332 = mf3_2r_clip_w + 3 * 7 mm"
equation "d333 = mf3_2r_clip_h"
equation "d334 = mf3_2r_key_h"
equation "d335 = mf3_2r_key_w"
equation "d336 = d332 + 3 mm"
equation "d350 = d349"
equation "d351 = d349"
equation "d352 = d349"
equation "d380 = d221"
equation "d381 = d221"
equation "d382 = d221"
equation "d384 = d221"
equation "d385 = d221"
